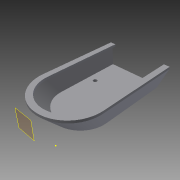
# Autodesk Inventor part: Robot Cover 1
Saved by Autodesk Inventor 2015 SP1 (Build 190203100, 203)
## iProperties
Created: 2017-06-09
Part Number: Robot Cover 1
Material: Generic
Document SubType Name: Modeling
Designer: 0301546
Density: 1 g/cm^3
Appearance: Default
Author: 0301546
Autodesk Inventor part; units mm, degrees
ref_plane "YZ Plane" through (0, 0, 0) normal (1, 0, 0) x (0, 1, 0)
ref_plane "XZ Plane" through (0, 0, 0) normal (0, 1, 0) x (-1, 0, 0)
sketch "Sketch1" plane through (0, 0, 0) normal (0, 1, 0) x (-1, 0, 0)
  line L0 (0, 0) -> (80, 0)
  line L1 (80, 0) -> (80, 100)
  line L2 (80, 100) -> (0, 100)
  line L3 (0, 100) -> (0, 0)
  arc A0 (80, 100) -> (0, 100) centre (40, 100) ccw
  dimension "d0" = 80
  dimension "d1" = 100
  constraints: 8 end point, 2 parallel, 2 point on circle, 1 centre point, 1 horizontal, 1 midpoint, 1 perpendicular
  measures "d0" distance of L0.start L0.end
  measures "d1" distance of L0.end L1.end
extrude "Extrusion1" add sketch "Sketch1" along normal blind 3
sketch3d "3D Sketch1"
ref_plane "Work Plane1" through (-7, -20, 0) normal (0, -1, 0.0000001) x (0, 0.0000001, 1)
sketch "Sketch8" plane through (-7, -20, 0) normal (0, -1, 0.0000001) x (0, 0.0000001, 1)
  line L0 (7.000002, 0) -> (7.000002, 66)
  line L1 (7.000002, 66) -> (87.000002, 66)
  line L2 (87.000002, 66) -> (87.000002, 0)
  line L3 (87.000002, 0) -> (7.000002, 0)
  line L4 (0.000002, -7) -> (0.000002, 73)
  line L5 (100.000002, -7) -> (0.000002, -7)
  line L6 (0.000002, 73) -> (100.000002, 73)
  line L7 (87.000002, 0) -> (87.000002, -7)
  line L8 (87.000002, 66) -> (87.000002, 73)
  line L9 (7.000002, 66) -> (0.000002, 66)
  arc A0 (87.000002, 0) -> (87.000002, 66) centre (87.000002, 33) ccw
  dimension "d24" = 7
  dimension "d25" = 7
  dimension "d26" = 7
  dimension "d27" = 80
  constraints: 14 end point, 4 parallel, 3 perpendicular, 3 point on line, 2 point on circle, 1 centre point, 1 collinear, 1 midpoint
  measures "d24" distance of L1.end L8.end
  measures "d25" distance of L2.end L7.end
  measures "d26" distance of L0.end L9.end
  measures "d27" distance of L0.end L1.end
extrude "Extrusion3" add sketch "Sketch8" along normal blind 3 contours L0 L1 L2 L3 | L2 A0
sketch "Sketch11" plane through (-7, -20, 0) normal (0, 1, -0.0000001) x (1, 0, 0)
  arc A0 (-66, -87.000002) -> (0, -87.000002) centre (-33, -87.000002) ccw
  line L0 (0, -87.000002) -> (0, -7.000002)
  line L1 (0, -87.000002) -> (-3, -87.000002)
  arc A1 (-66, -87.000002) -> (0, -87.000002) centre (-33, -87.000002) ccw
  line L2 (-3, -87.000002) -> (-3, -10.000002)
  line L3 (-63, -87.000002) -> (-63, -10.000002)
  line L4 (-66, -7.000002) -> (0, -7.000002)
  line L5 (-66, -87.000002) -> (-66, -7.000002)
  arc A2 (-63, -87.000002) -> (-3, -87.000002) centre (-33, -87.000002) ccw
  line L6 (-3, -87.000002) -> (-63, -87.000002)
  line L7 (-63, -87.000002) -> (-66, -87.000002)
  line L8 (0, -7.000002) -> (0, -87.000002)
  line L9 (-66, -87.000002) -> (-66, -7.000002)
  line L10 (-66, -7.000002) -> (0, -7.000002)
  line L11 (-66, -7.000002) -> (0, -7.000002)
  line L12 (-3, -10.000002) -> (-3, -7.000002)
  line L13 (-63, -10.000002) -> (-63, -7.000002)
  line L14 (-3, -7.000002) -> (-3, 12.999998)
  line L15 (-3, 12.999998) -> (-63, 12.999998)
  line L16 (-63, 12.999998) -> (-63, -7.000002)
  dimension "d63" = 3
  dimension "d66" = 20
  constraints: 26 end point, 5 collinear, 4 point on circle, 3 horizontal, 3 point on line, 2 centre point, 2 coincident, 2 parallel, 2 tangent, 1 perpendicular, 1 vertical
  measures "d63" distance of L0.start L1.end
  measures "d66" distance of L15.end L13.end
loft "Loft1" add section 1 edges at (-40, 0, 140) (-80, 0, 50) (-40, 0, 0) (0, 0, 50) section 2 edges at (-40, -22.999985, 120.000003) (-73, -22.999994, 47.000003) (-40, -22.999999, 7.000003) (-7, -22.999994, 47.000003)
sketch "Sketch12" plane through (0, 0, 0) normal (0, -1, 0) x (1, 0, 0)
  line L0 (-77, 3) -> (-3, 3)
  line L1 (-3, 3) -> (-3, 100)
  line L2 (-3, 100) -> (-77, 100)
  line L3 (-77, 100) -> (-77, 3)
  line L4 (-77, 3) -> (-77, 0)
  line L5 (0, 0) -> (-80, 0) projected
  line L6 (-3, 3) -> (0, 3)
  line L7 (-77, 3) -> (-80, 3)
  line L8 (-80, 0) -> (-80, 100) projected
  line L9 (0, 100) -> (0, 0) projected
  arc A0 (0, 100) -> (-80, 100) centre (-40, 100) ccw projected
  circle A1 centre (-40, 100) radius 37
  line L10 (-3, 3) -> (-3, 0)
  line L11 (-77, -17) -> (-3, -17)
  line L12 (-3, -17) -> (-3, 3)
  line L13 (-77, -17) -> (-77, 3)
  dimension "d49" = 3
  dimension "d50" = 3
  dimension "d51" = 3
  dimension "d65" = 20
  constraints: 22 end point, 4 collinear, 4 parallel, 4 point on line, 2 perpendicular, 1 coincident, 1 horizontal, 1 horizontal alignment, 1 midpoint, 2 other
  measures "d49" distance of L0.end L6.end
  measures "d50" distance of L0.start L4.end
  measures "d51" distance of L0.start L7.end
  measures "d65" distance of L11.end L0.end
loft "Loft2" cut profiles "Sketch12", "Sketch11" contours L3 A1 L1 L0 | L0 L10 L5 L4 | A1 L2 | L2 A1 | L5 L12 L11 L13 / L6 A2 | L3 L13 L4 L12 L2 L6 | L16 L15 L14 L4
sketch "Sketch13" plane through (0, 3, 0) normal (0, 1, 0) x (1, 0, 0)
  line L0 (-73, -100) -> (-73, -7)
  line L1 (-73, -7) -> (-7, -7)
  line L2 (-7, -7) -> (-7, -100)
  line L3 (-7, -100) -> (-73, -100)
  line L4 (-73, -7) -> (-73, 0)
  line L5 (-73, -7) -> (-80, -7)
  line L6 (-80, 0) -> (-80, -100) projected
  line L7 (-7, -7) -> (0, -7)
  line L8 (-80, 0) -> (-80, -100) projected
  line L9 (0, -100) -> (0, 0) projected
  line L10 (0, 0) -> (-80, 0) projected
  circle A0 centre (-40, -100) radius 33
  line L11 (-7, -7) -> (-7, 0)
  dimension "d57" = 7
  dimension "d58" = 7
  dimension "d59" = 7
  dimension "d60" = 93
  constraints: 16 end point, 6 point on line, 3 parallel, 2 perpendicular, 2 vertical, 1 horizontal, 1 horizontal alignment, 1 midpoint, 2 other
  measures "d57" distance of L0.end L5.end
  measures "d58" distance of L1.end L7.end
  measures "d59" distance of L0.end L4.end
  measures "d60" distance of L0.start L0.end
extrude "Extrusion4" cut sketch "Sketch13" against normal blind 3 contours A0 L3 | L0 L1 L2 A0 | L3 A0 | L4 L10 L11 L1
sketch3d "3D Sketch2"
ref_plane "Work Plane2" through (-40, -4.999994, 150.000001) normal (0, 0.0000001, 1) x (1, 0, 0)
sketch "Sketch14" plane through (-40, -4.999994, 150.000001) normal (0, 0.0000001, 1) x (1, 0, 0)
  ellipse E0 centre (0, 5) end of major axis (-37, 5) minor radius 0.000005 (-37, 5) -> (37, 5) ccw
  line L0 (0, 5) -> (0, 0)
  line L1 (0, 0) -> (-2.7, 0)
  circle A0 centre (0, 0) radius 2.7
  point P0 (40, 5.000012)
  dimension "d76" = 5
  dimension "d77" = 2.7
  constraints: 4 end point, 1 coincident, 1 horizontal, 1 horizontal alignment, 1 vertical, 3 other
  measures "d76" distance of L0.start L0.end
  measures "d77" distance of L0.end L1.end
extrude "Extrusion5" cut sketch "Sketch14" against normal blind 21.75
sketch "Sketch15" plane through (-40, -4.999994, 150.000001) normal (0, 0.0000001, 1) x (1, 0, 0)
  point P0 (40, 5.000012)
sketch "Sketch16" plane through (-7, -23, 0) normal (0, -1, 0.0000001) x (1, 0, 0)
  line L0 (0, 87.000002) -> (0, 7.000002)
  line L1 (0, 7.000002) -> (-66, 7.000002)
  line L2 (-66, 7.000002) -> (-66, 87.000002)
  line L3 (-66, 87.000002) -> (-66, 7.000002)
  line L4 (-66, 7.000002) -> (0, 7.000002)
  line L5 (0, 7.000002) -> (0, 87.000002)
  line L6 (0, 47.000002) -> (-13, 47.000002)
  line L7 (-66, 47.000002) -> (-53, 47.000002)
  circle A0 centre (-13, 47.000002) radius 2.7
  circle A1 centre (-53, 47.000002) radius 2.7
  point P0 (7, 0.000002)
  dimension "d78" = 13
  dimension "d79" = 13
  dimension "d80" = 5.4
  dimension "d81" = 5.4
  constraints: 10 end point, 3 midpoint, 2 centre point, 2 coincident, 2 collinear, 2 horizontal, 1 perpendicular, 1 vertical
  measures "d78" distance of L6.start L6.end
  measures "d79" distance of L7.start L7.end
  measures "d80" diameter of A0
  measures "d81" diameter of A1
extrude "Extrusion6" cut sketch "Sketch16" against normal blind 21.75
sketch "Sketch18" plane through (-7, -23, 0) normal (0, -1, 0.0000001) x (1, 0, 0)
  arc A0 (0, 87.000002) -> (-66, 87.000002) centre (-33, 87.000002) ccw
  circle A1 centre (-33, 87.000002) radius 33
  line L0 (-2.41471, 89.14761) -> (-2.446153, 88.174292)
  line L1 (-2.446153, 88.174292) -> (-7.698114, 88.343958)
  line L2 (-7.698114, 88.343958) -> (-4.18744, 86.326392)
  line L3 (-4.18744, 86.326392) -> (-4.206593, 85.733508)
  line L4 (-4.206593, 85.733508) -> (-7.839688, 83.96156)
  line L5 (-7.839688, 83.96156) -> (-2.587727, 83.791895)
  line L6 (-2.587727, 83.791895) -> (-2.617096, 82.882806)
  line L7 (-2.617096, 82.882806) -> (-8.713915, 83.079765)
  line L8 (-8.713915, 83.079765) -> (-8.67114, 84.403872)
  line L9 (-8.67114, 84.403872) -> (-5.217825, 86.122278)
  line L10 (-5.217825, 86.122278) -> (-8.555103, 87.995758)
  line L11 (-8.555103, 87.995758) -> (-8.51153, 89.344569)
  line L12 (-8.51153, 89.344569) -> (-2.41471, 89.14761)
  spline S0 degree 2 poles (-5.708587, 94.553393) (-4.57126, 94.764353) (-3.088451, 93.681946) (-2.886507, 92.593223) knots 0 0 0 1 2 2 2
  spline S1 degree 2 poles (-2.886507, 92.593223) (-2.67735, 91.465617) (-3.716719, 89.940515) (-4.815163, 89.736767) knots 0 0 0 1 2 2 2
  spline S2 degree 2 poles (-4.815163, 89.736767) (-5.942768, 89.527611) (-7.438003, 90.622796) (-7.639947, 91.711519) knots 0 0 0 1 2 2 2
  spline S3 degree 2 poles (-7.639947, 91.711519) (-7.841892, 92.800241) (-6.841053, 94.343335) (-5.708587, 94.553393) knots 0 0 0 1 2 2 2
  spline S4 degree 2 poles (-5.53459, 93.615342) (-6.409456, 93.453065) (-7.118479, 92.532218) (-6.987756, 91.827464) knots 0 0 0 1 2 2 2
  spline S5 degree 2 poles (-6.987756, 91.827464) (-6.857033, 91.122711) (-5.864026, 90.512542) (-4.989159, 90.674819) knots 0 0 0 1 2 2 2
  spline S6 degree 2 poles (-4.989159, 90.674819) (-4.138595, 90.832588) (-3.406171, 91.762803) (-3.536894, 92.467557) knots 0 0 0 1 2 2 2
  spline S7 degree 2 poles (-3.536894, 92.467557) (-3.666716, 93.16745) (-4.669444, 93.775816) (-5.53459, 93.615342) knots 0 0 0 1 2 2 2
  line L13 (-5.265037, 99.868285) -> (-4.935567, 99.004601)
  line L14 (-4.935567, 99.004601) -> (-5.406668, 98.82489)
  spline S8 degree 2 poles (-5.406668, 98.82489) (-4.964173, 98.538685) (-4.389111, 97.9327) (-4.221733, 97.49393) knots 0 0 0 1 2 2 2
  spline S9 degree 2 poles (-4.221733, 97.49393) (-4.093117, 97.156769) (-4.052343, 96.495109) (-4.166375, 96.197655) knots 0 0 0 1 2 2 2
  spline S10 degree 2 poles (-4.166375, 96.197655) (-4.282168, 95.904819) (-4.79383, 95.429226) (-5.227982, 95.263611) knots 0 0 0 1 2 2 2
  line L15 (-5.227982, 95.263611) -> (-8.003781, 94.204728)
  line L16 (-8.003781, 94.204728) -> (-8.33325, 95.068413)
  line L17 (-8.33325, 95.068413) -> (-5.894612, 95.998679)
  spline S11 degree 2 poles (-5.894612, 95.998679) (-5.552833, 96.129057) (-5.12773, 96.360001) (-5.001982, 96.529656) knots 0 0 0 1 2 2 2
  spline S12 degree 2 poles (-5.001982, 96.529656) (-4.876234, 96.699312) (-4.861245, 97.117707) (-4.991623, 97.459486) knots 0 0 0 1 2 2 2
  spline S13 degree 2 poles (-4.991623, 97.459486) (-5.11143, 97.773553) (-5.68473, 98.37492) (-6.016328, 98.592324) knots 0 0 0 1 2 2 2
  line L18 (-6.016328, 98.592324) -> (-9.212422, 97.373111)
  line L19 (-9.212422, 97.373111) -> (-9.541892, 98.236796)
  line L20 (-9.541892, 98.236796) -> (-5.265037, 99.868285)
  line L21 (-8.098287, 104.745318) -> (-7.616799, 103.956223)
  line L22 (-7.616799, 103.956223) -> (-9.844832, 102.596729)
  spline S14 degree 2 poles (-9.844832, 102.596729) (-10.114896, 102.431942) (-10.540448, 102.085418) (-10.625629, 101.911834) knots 0 0 0 1 2 2 2
  spline S15 degree 2 poles (-10.625629, 101.911834) (-10.7141, 101.724662) (-10.649013, 101.295318) (-10.466203, 100.995715) knots 0 0 0 1 2 2 2
  spline S16 degree 2 poles (-10.466203, 100.995715) (-10.288541, 100.704552) (-9.645846, 100.239665) (-9.252047, 100.068802) knots 0 0 0 1 2 2 2
  line L23 (-9.252047, 100.068802) -> (-6.331974, 101.850563)
  line L24 (-6.331974, 101.850563) -> (-5.850487, 101.061469)
  line L25 (-5.850487, 101.061469) -> (-9.757984, 98.677204)
  line L26 (-9.757984, 98.677204) -> (-10.239471, 99.466299)
  line L27 (-10.239471, 99.466299) -> (-9.804836, 99.731504)
  spline S17 degree 2 poles (-9.804836, 99.731504) (-10.286964, 99.923751) (-10.98516, 100.441635) (-11.216892, 100.821413) knots 0 0 0 1 2 2 2
  spline S18 degree 2 poles (-11.216892, 100.821413) (-11.639159, 101.513454) (-11.355941, 102.757573) (-10.634362, 103.197864) knots 0 0 0 1 2 2 2
  line L28 (-10.634362, 103.197864) -> (-8.098287, 104.745318)
  spline S19 degree 2 poles (-9.913482, 107.077714) (-9.429309, 106.496682) (-9.438824, 105.388437) (-10.035046, 104.891606) knots 0 0 0 1 2 2 2
  line L29 (-10.035046, 104.891606) -> (-11.98321, 103.2682)
  line L30 (-11.98321, 103.2682) -> (-11.584479, 102.789704)
  line L31 (-11.584479, 102.789704) -> (-12.074368, 102.381479)
  line L32 (-12.074368, 102.381479) -> (-12.473099, 102.859976)
  line L33 (-12.473099, 102.859976) -> (-13.483258, 102.01821)
  line L34 (-13.483258, 102.01821) -> (-14.075026, 102.72836)
  line L35 (-14.075026, 102.72836) -> (-13.064867, 103.570125)
  line L36 (-13.064867, 103.570125) -> (-14.153466, 104.876496)
  line L37 (-14.153466, 104.876496) -> (-13.663577, 105.284721)
  line L38 (-13.663577, 105.284721) -> (-12.574978, 103.97835)
  line L39 (-12.574978, 103.97835) -> (-10.90024, 105.373909)
  spline S20 degree 2 poles (-10.90024, 105.373909) (-10.634409, 105.595426) (-10.360982, 105.86188) (-10.298952, 106.042262) knots 0 0 0 1 2 2 2
  spline S21 degree 2 poles (-10.298952, 106.042262) (-10.242619, 106.198592) (-10.369828, 106.575183) (-10.575523, 106.822026) knots 0 0 0 1 2 2 2
  spline S22 degree 2 poles (-10.575523, 106.822026) (-10.721092, 106.996716) (-11.077421, 107.246726) (-11.164131, 107.296729) knots 0 0 0 1 2 2 2
  line L40 (-11.164131, 107.296729) -> (-11.19894, 107.338502)
  line L41 (-11.19894, 107.338502) -> (-10.667278, 107.781537)
  spline S23 degree 2 poles (-10.667278, 107.781537) (-10.453987, 107.618239) (-10.059051, 107.252403) (-9.913482, 107.077714) knots 0 0 0 1 2 2 2
  line L42 (-18.059872, 113.792399) -> (-17.031002, 113.064131)
  line L43 (-17.031002, 113.064131) -> (-16.540962, 109.743609)
  line L44 (-16.540962, 109.743609) -> (-15.633136, 109.101019)
  line L45 (-15.633136, 109.101019) -> (-14.230862, 111.082098)
  line L46 (-14.230862, 111.082098) -> (-13.43601, 110.519475)
  line L47 (-13.43601, 110.519475) -> (-16.960258, 105.540552)
  line L48 (-16.960258, 105.540552) -> (-18.501545, 106.631526)
  spline S24 degree 2 poles (-18.501545, 106.631526) (-19.013963, 106.994233) (-19.642259, 107.578257) (-19.832987, 107.967626) knots 0 0 0 1 2 2 2
  spline S25 degree 2 poles (-19.832987, 107.967626) (-20.02775, 108.359852) (-20.016751, 109.145444) (-19.739723, 109.536818) knots 0 0 0 1 2 2 2
  spline S26 degree 2 poles (-19.739723, 109.536818) (-19.354169, 110.081514) (-18.16579, 110.348647) (-17.467189, 110.120632) knots 0 0 0 1 2 2 2
  line L49 (-17.467189, 110.120632) -> (-18.059872, 113.792399)
  spline S27 degree 2 poles (-18.875465, 109.0038) (-19.029686, 108.785922) (-19.081131, 108.319661) (-18.968607, 108.076492) knots 0 0 0 1 2 2 2
  spline S28 degree 2 poles (-18.968607, 108.076492) (-18.864833, 107.863741) (-18.4672, 107.467214) (-18.136348, 107.233025) knots 0 0 0 1 2 2 2
  line L50 (-18.136348, 107.233025) -> (-17.349565, 106.676114)
  line L51 (-17.349565, 106.676114) -> (-16.024402, 108.548254)
  line L52 (-16.024402, 108.548254) -> (-16.722419, 109.042334)
  spline S29 degree 2 poles (-16.722419, 109.042334) (-17.065376, 109.28509) (-17.681471, 109.569774) (-17.982488, 109.546648) knots 0 0 0 1 2 2 2
  spline S30 degree 2 poles (-17.982488, 109.546648) (-18.253086, 109.532271) (-18.692684, 109.262026) (-18.875465, 109.0038) knots 0 0 0 1 2 2 2
  spline S31 degree 2 poles (-23.608454, 113.714677) (-23.131869, 114.76866) (-21.396378, 115.367327) (-20.387436, 114.911109) knots 0 0 0 1 2 2 2
  spline S32 degree 2 poles (-20.387436, 114.911109) (-19.342461, 114.438597) (-18.684496, 112.714269) (-19.144787, 111.696318) knots 0 0 0 1 2 2 2
  spline S33 degree 2 poles (-19.144787, 111.696318) (-19.617299, 110.651343) (-21.370376, 110.049778) (-22.379317, 110.505997) knots 0 0 0 1 2 2 2
  spline S34 degree 2 poles (-22.379317, 110.505997) (-23.388259, 110.962215) (-24.083002, 112.665197) (-23.608454, 113.714677) knots 0 0 0 1 2 2 2
  spline S35 degree 2 poles (-22.739142, 113.321596) (-23.105746, 112.510839) (-22.755007, 111.402843) (-22.101897, 111.107523) knots 0 0 0 1 2 2 2
  spline S36 degree 2 poles (-22.101897, 111.107523) (-21.448787, 110.812203) (-20.380703, 111.278642) (-20.014099, 112.089399) knots 0 0 0 1 2 2 2
  spline S37 degree 2 poles (-20.014099, 112.089399) (-19.657678, 112.877635) (-20.002739, 114.010189) (-20.655848, 114.305508) knots 0 0 0 1 2 2 2
  spline S38 degree 2 poles (-20.655848, 114.305508) (-21.304454, 114.598792) (-22.376612, 114.123344) (-22.739142, 113.321596) knots 0 0 0 1 2 2 2
  line L53 (-28.900006, 112.716014) -> (-24.472723, 118.039089)
  line L54 (-24.472723, 118.039089) -> (-23.515652, 117.791192)
  line L55 (-23.515652, 117.791192) -> (-24.946378, 116.190702)
  line L56 (-24.946378, 116.190702) -> (-24.105079, 111.474051)
  line L57 (-24.105079, 111.474051) -> (-25.066936, 111.723187)
  line L58 (-25.066936, 111.723187) -> (-25.671399, 115.382745)
  line L59 (-25.671399, 115.382745) -> (-27.966862, 112.474314)
  line L60 (-27.966862, 112.474314) -> (-28.900006, 112.716014)
  spline S39 degree 2 poles (-31.529156, 116.999221) (-31.409984, 117.0585) (-31.014623, 117.272795) (-30.831001, 117.33153) knots 0 0 0 1 2 2 2
  spline S40 degree 2 poles (-30.831001, 117.33153) (-30.575479, 117.418853) (-30.112671, 117.493433) (-29.703868, 117.458515) knots 0 0 0 1 2 2 2
  spline S41 degree 2 poles (-29.703868, 117.458515) (-29.36402, 117.429488) (-28.776292, 117.165954) (-28.561208, 116.954093) knots 0 0 0 1 2 2 2
  spline S42 degree 2 poles (-28.561208, 116.954093) (-28.360479, 116.74842) (-28.141628, 116.174064) (-28.167711, 115.868693) knots 0 0 0 1 2 2 2
  spline S43 degree 2 poles (-28.167711, 115.868693) (-28.208097, 115.395861) (-28.743068, 114.766821) (-29.281561, 114.619326) knots 0 0 0 1 2 2 2
  spline S44 degree 2 poles (-29.281561, 114.619326) (-29.754763, 114.481138) (-31.017158, 114.455008) (-31.744128, 114.482372) knots 0 0 0 1 2 2 2
  line L61 (-31.744128, 114.482372) -> (-31.756748, 114.334612)
  spline S45 degree 2 poles (-31.756748, 114.334612) (-31.779466, 114.068643) (-31.610638, 113.721818) (-31.446244, 113.613512) knots 0 0 0 1 2 2 2
  spline S46 degree 2 poles (-31.446244, 113.613512) (-31.276925, 113.504786) (-30.769738, 113.401931) (-30.503769, 113.379213) knots 0 0 0 1 2 2 2
  spline S47 degree 2 poles (-30.503769, 113.379213) (-30.183622, 113.351869) (-29.308226, 113.435859) (-28.86668, 113.551945) knots 0 0 0 1 2 2 2
  line L62 (-28.86668, 113.551945) -> (-28.812501, 113.547317)
  line L63 (-28.812501, 113.547317) -> (-28.87939, 112.764188)
  spline S48 degree 2 poles (-28.87939, 112.764188) (-29.140556, 112.72696) (-30.103768, 112.660392) (-30.56675, 112.699937) knots 0 0 0 1 2 2 2
  spline S49 degree 2 poles (-30.56675, 112.699937) (-31.133164, 112.748316) (-31.893822, 112.962124) (-32.187711, 113.180716) knots 0 0 0 1 2 2 2
  spline S50 degree 2 poles (-32.187711, 113.180716) (-32.467246, 113.39312) (-32.711863, 114.014328) (-32.675263, 114.442832) knots 0 0 0 1 2 2 2
  line L64 (-32.675263, 114.442832) -> (-32.408967, 117.560573)
  line L65 (-32.408967, 117.560573) -> (-31.487929, 117.481904)
  line L66 (-31.487929, 117.481904) -> (-31.529156, 116.999221)
  line L67 (-31.583846, 116.358927) -> (-31.691962, 115.093114)
  spline S51 degree 2 poles (-31.691962, 115.093114) (-31.364786, 115.089975) (-30.352865, 115.087886) (-30.040763, 115.140609) knots 0 0 0 1 2 2 2
  spline S52 degree 2 poles (-30.040763, 115.140609) (-29.66337, 115.202638) (-29.152377, 115.550934) (-29.122929, 115.895707) knots 0 0 0 1 2 2 2
  spline S53 degree 2 poles (-29.122929, 115.895707) (-29.089274, 116.289735) (-29.58221, 116.733701) (-30.08952, 116.777032) knots 0 0 0 1 2 2 2
  spline S54 degree 2 poles (-30.08952, 116.777032) (-30.527875, 116.814473) (-31.258702, 116.564335) (-31.583846, 116.358927) knots 0 0 0 1 2 2 2
  line L68 (-34.644676, 117.459134) -> (-33.720979, 117.494983)
  line L69 (-33.720979, 117.494983) -> (-33.47387, 111.127896)
  line L70 (-33.47387, 111.127896) -> (-34.397567, 111.092047)
  line L71 (-34.397567, 111.092047) -> (-34.644676, 117.459134)
  line L72 (-39.181257, 116.939493) -> (-37.544054, 111.063307)
  line L73 (-37.544054, 111.063307) -> (-41.953574, 109.834741)
  line L74 (-41.953574, 109.834741) -> (-42.147279, 110.529979)
  line L75 (-42.147279, 110.529979) -> (-38.675853, 111.497176)
  line L76 (-38.675853, 111.497176) -> (-39.124293, 113.106699)
  line L77 (-39.124293, 113.106699) -> (-42.357624, 112.205839)
  line L78 (-42.357624, 112.205839) -> (-42.551329, 112.901076)
  line L79 (-42.551329, 112.901076) -> (-39.317998, 113.801936)
  line L80 (-39.317998, 113.801936) -> (-39.925647, 115.982887)
  line L81 (-39.925647, 115.982887) -> (-43.397073, 115.01569)
  line L82 (-43.397073, 115.01569) -> (-43.590778, 115.710927)
  line L83 (-43.590778, 115.710927) -> (-39.181257, 116.939493)
  line L84 (-45.349615, 114.891769) -> (-44.498796, 115.253167)
  line L85 (-44.498796, 115.253167) -> (-42.007662, 109.388433)
  line L86 (-42.007662, 109.388433) -> (-42.85848, 109.027035)
  line L87 (-42.85848, 109.027035) -> (-45.349615, 114.891769)
  spline S55 degree 2 poles (-48.711561, 113.265994) (-47.578612, 113.923598) (-45.708056, 113.586141) (-45.137306, 112.602828) knots 0 0 0 1 2 2 2
  spline S56 degree 2 poles (-45.137306, 112.602828) (-44.576481, 111.636615) (-45.12561, 109.786088) (-46.104649, 109.217818) knots 0 0 0 1 2 2 2
  spline S57 degree 2 poles (-46.104649, 109.217818) (-46.549277, 108.95974) (-47.348847, 108.781422) (-47.736885, 108.85912) knots 0 0 0 1 2 2 2
  spline S58 degree 2 poles (-47.736885, 108.85912) (-48.120647, 108.9393) (-48.773938, 109.4346) (-49.049387, 109.909155) knots 0 0 0 1 2 2 2
  line L88 (-49.049387, 109.909155) -> (-49.260317, 110.272554)
  line L89 (-49.260317, 110.272554) -> (-45.976905, 112.178366)
  spline S59 degree 2 poles (-45.976905, 112.178366) (-46.37643, 112.866685) (-47.630175, 113.116341) (-48.365523, 112.689519) knots 0 0 0 1 2 2 2
  spline S60 degree 2 poles (-48.365523, 112.689519) (-48.63059, 112.535664) (-49.077997, 112.144513) (-49.234268, 111.950926) knots 0 0 0 1 2 2 2
  spline S61 degree 2 poles (-49.234268, 111.950926) (-49.402676, 111.738863) (-49.610817, 111.418003) (-49.669444, 111.292523) knots 0 0 0 1 2 2 2
  line L90 (-49.669444, 111.292523) -> (-49.716472, 111.265227)
  line L91 (-49.716472, 111.265227) -> (-50.138331, 111.992024)
  spline S62 degree 2 poles (-50.138331, 111.992024) (-50.024544, 112.120942) (-49.689251, 112.498459) (-49.544849, 112.633716) knots 0 0 0 1 2 2 2
  spline S63 degree 2 poles (-49.544849, 112.633716) (-49.346244, 112.823297) (-48.998004, 113.099731) (-48.711561, 113.265994) knots 0 0 0 1 2 2 2
  spline S64 degree 2 poles (-48.186915, 110.215434) (-48.022029, 109.951054) (-47.656919, 109.637138) (-47.456009, 109.576568) knots 0 0 0 1 2 2 2
  spline S65 degree 2 poles (-47.456009, 109.576568) (-47.228071, 109.508824) (-46.700177, 109.603754) (-46.375256, 109.79235) knots 0 0 0 1 2 2 2
  spline S66 degree 2 poles (-46.375256, 109.79235) (-46.058885, 109.975983) (-45.706073, 110.392247) (-45.611571, 110.652863) knots 0 0 0 1 2 2 2
  spline S67 degree 2 poles (-45.611571, 110.652863) (-45.528101, 110.912791) (-45.560845, 111.402477) (-45.681603, 111.669608) knots 0 0 0 1 2 2 2
  line L92 (-45.681603, 111.669608) -> (-48.186915, 110.215434)
  spline S68 degree 2 poles (-52.84998, 110.299114) (-52.414795, 110.657141) (-51.500375, 111.031768) (-51.052355, 111.016284) knots 0 0 0 1 2 2 2
  spline S69 degree 2 poles (-51.052355, 111.016284) (-50.603658, 111.007758) (-49.745764, 110.548534) (-49.362612, 110.08281) knots 0 0 0 1 2 2 2
  spline S70 degree 2 poles (-49.362612, 110.08281) (-48.979459, 109.617086) (-48.718191, 108.69262) (-48.781704, 108.256296) knots 0 0 0 1 2 2 2
  spline S71 degree 2 poles (-48.781704, 108.256296) (-48.842077, 107.816155) (-49.382333, 106.955607) (-49.809883, 106.603861) knots 0 0 0 1 2 2 2
  spline S72 degree 2 poles (-49.809883, 106.603861) (-50.161085, 106.314926) (-50.941273, 105.948314) (-51.284976, 105.844782) knots 0 0 0 1 2 2 2
  line L93 (-51.284976, 105.844782) -> (-51.83458, 106.512828)
  line L94 (-51.83458, 106.512828) -> (-51.792589, 106.547375)
  spline S73 degree 2 poles (-51.792589, 106.547375) (-51.672272, 106.556743) (-51.322531, 106.614033) (-51.091077, 106.682829) knots 0 0 0 1 2 2 2
  spline S74 degree 2 poles (-51.091077, 106.682829) (-50.891948, 106.744234) (-50.412605, 106.978561) (-50.225552, 107.13245) knots 0 0 0 1 2 2 2
  spline S75 degree 2 poles (-50.225552, 107.13245) (-49.672028, 107.587837) (-49.574892, 108.839167) (-50.099372, 109.476675) knots 0 0 0 1 2 2 2
  spline S76 degree 2 poles (-50.099372, 109.476675) (-50.611289, 110.098913) (-51.834978, 110.263597) (-52.411406, 109.789368) knots 0 0 0 1 2 2 2
  spline S77 degree 2 poles (-52.411406, 109.789368) (-52.758791, 109.503573) (-53.190806, 108.744878) (-53.281231, 108.356827) knots 0 0 0 1 2 2 2
  line L95 (-53.281231, 108.356827) -> (-53.323222, 108.322281)
  line L96 (-53.323222, 108.322281) -> (-53.872827, 108.990327)
  spline S78 degree 2 poles (-53.872827, 108.990327) (-53.800486, 109.120256) (-53.580999, 109.499265) (-53.473191, 109.632767) knots 0 0 0 1 2 2 2
  spline S79 degree 2 poles (-53.473191, 109.632767) (-53.327643, 109.829324) (-53.079024, 110.110678) (-52.84998, 110.299114) knots 0 0 0 1 2 2 2
  spline S80 degree 2 poles (-55.795106, 107.407965) (-55.278857, 107.960693) (-54.178045, 108.089192) (-53.610867, 107.559446) knots 0 0 0 1 2 2 2
  line L97 (-53.610867, 107.559446) -> (-51.757602, 105.828494)
  line L98 (-51.757602, 105.828494) -> (-51.332456, 106.283681)
  line L99 (-51.332456, 106.283681) -> (-50.866431, 105.848412)
  line L100 (-50.866431, 105.848412) -> (-51.291577, 105.393225)
  line L101 (-51.291577, 105.393225) -> (-50.330625, 104.495694)
  line L102 (-50.330625, 104.495694) -> (-50.961596, 103.820137)
  line L103 (-50.961596, 103.820137) -> (-51.922548, 104.717668)
  line L104 (-51.922548, 104.717668) -> (-53.083265, 103.474933)
  line L105 (-53.083265, 103.474933) -> (-53.54929, 103.910202)
  line L106 (-53.54929, 103.910202) -> (-52.388574, 105.152937)
  line L107 (-52.388574, 105.152937) -> (-53.981731, 106.640949)
  spline S81 degree 2 poles (-53.981731, 106.640949) (-54.234613, 106.877142) (-54.533028, 107.115278) (-54.719728, 107.154373) knots 0 0 0 1 2 2 2
  spline S82 degree 2 poles (-54.719728, 107.154373) (-54.881854, 107.19081) (-55.239683, 107.017716) (-55.459004, 106.782897) knots 0 0 0 1 2 2 2
  spline S83 degree 2 poles (-55.459004, 106.782897) (-55.614216, 106.616718) (-55.817932, 106.23204) (-55.856753, 106.139782) knots 0 0 0 1 2 2 2
  line L108 (-55.856753, 106.139782) -> (-55.893869, 106.100043)
  line L109 (-55.893869, 106.100043) -> (-56.399633, 106.572428)
  spline S84 degree 2 poles (-56.399633, 106.572428) (-56.264153, 106.804386) (-55.950318, 107.241785) (-55.795106, 107.407965) knots 0 0 0 1 2 2 2
  line L110 (-55.553037, 101.488777) -> (-55.523642, 101.528521)
  spline S85 degree 2 poles (-55.523642, 101.528521) (-55.442041, 101.597284) (-55.298875, 101.774224) (-55.201872, 101.905377) knots 0 0 0 1 2 2 2
  spline S86 degree 2 poles (-55.201872, 101.905377) (-54.97847, 102.207426) (-54.762012, 102.9573) (-54.77968, 103.382313) knots 0 0 0 1 2 2 2
  line L111 (-54.77968, 103.382313) -> (-57.390816, 105.313563)
  line L112 (-57.390816, 105.313563) -> (-56.841129, 106.056763)
  line L113 (-56.841129, 106.056763) -> (-53.160899, 103.334788)
  line L114 (-53.160899, 103.334788) -> (-53.710585, 102.591588)
  line L115 (-53.710585, 102.591588) -> (-54.259042, 102.997239)
  spline S87 degree 2 poles (-54.259042, 102.997239) (-54.256822, 102.368455) (-54.457217, 101.582108) (-54.668861, 101.295956) knots 0 0 0 1 2 2 2
  spline S88 degree 2 poles (-54.668861, 101.295956) (-54.751167, 101.184675) (-54.844361, 101.075298) (-54.909195, 101.012579) knots 0 0 0 1 2 2 2
  line L116 (-54.909195, 101.012579) -> (-55.553037, 101.488777)
  spline S89 degree 2 poles (-59.064586, 98.068529) (-60.086189, 98.611063) (-60.573474, 100.381058) (-60.054126, 101.359003) knots 0 0 0 1 2 2 2
  spline S90 degree 2 poles (-60.054126, 101.359003) (-59.516229, 102.371874) (-57.75361, 102.919047) (-56.766933, 102.395061) knots 0 0 0 1 2 2 2
  spline S91 degree 2 poles (-56.766933, 102.395061) (-55.754062, 101.857164) (-55.265001, 100.069435) (-55.784349, 99.09149) knots 0 0 0 1 2 2 2
  spline S92 degree 2 poles (-55.784349, 99.09149) (-56.303698, 98.113545) (-58.047349, 97.528314) (-59.064586, 98.068529) knots 0 0 0 1 2 2 2
  spline S93 degree 2 poles (-58.617112, 98.911133) (-57.831264, 98.4938) (-56.703237, 98.773493) (-56.367051, 99.406538) knots 0 0 0 1 2 2 2
  spline S94 degree 2 poles (-56.367051, 99.406538) (-56.030866, 100.039582) (-56.428559, 101.135123) (-57.214408, 101.552457) knots 0 0 0 1 2 2 2
  spline S95 degree 2 poles (-57.214408, 101.552457) (-57.978427, 101.958198) (-59.130601, 101.685731) (-59.466787, 101.052687) knots 0 0 0 1 2 2 2
  spline S96 degree 2 poles (-59.466787, 101.052687) (-59.800654, 100.424008) (-59.394229, 99.32383) (-58.617112, 98.911133) knots 0 0 0 1 2 2 2
  line L117 (-62.730862, 94.14615) -> (-62.45137, 95.027277)
  line L118 (-62.45137, 95.027277) -> (-59.963481, 94.238123)
  spline S97 degree 2 poles (-59.963481, 94.238123) (-59.661919, 94.142468) (-59.121189, 94.048739) (-58.93431, 94.098367) knots 0 0 0 1 2 2 2
  spline S98 degree 2 poles (-58.93431, 94.098367) (-58.735017, 94.15443) (-58.453748, 94.485278) (-58.347631, 94.819823) knots 0 0 0 1 2 2 2
  spline S99 degree 2 poles (-58.347631, 94.819823) (-58.244503, 95.144945) (-58.315439, 95.934974) (-58.444917, 96.34425) knots 0 0 0 1 2 2 2
  line L119 (-58.444917, 96.34425) -> (-61.705559, 97.37852)
  line L120 (-61.705559, 97.37852) -> (-61.426067, 98.259647)
  line L121 (-61.426067, 98.259647) -> (-57.062838, 96.875638)
  line L122 (-57.062838, 96.875638) -> (-57.34233, 95.994511)
  line L123 (-57.34233, 95.994511) -> (-57.827657, 96.148456)
  spline S100 degree 2 poles (-57.827657, 96.148456) (-57.656354, 95.658495) (-57.588989, 94.791809) (-57.723504, 94.367738) knots 0 0 0 1 2 2 2
  spline S101 degree 2 poles (-57.723504, 94.367738) (-57.96862, 93.594984) (-59.093267, 92.992311) (-59.899004, 93.247889) knots 0 0 0 1 2 2 2
  line L124 (-59.899004, 93.247889) -> (-62.730862, 94.14615)
  line L125 (-63.101039, 91.938733) -> (-62.937569, 92.848557)
  line L126 (-62.937569, 92.848557) -> (-58.432241, 92.039073)
  line L127 (-58.432241, 92.039073) -> (-58.595711, 91.12925)
  line L128 (-58.595711, 91.12925) -> (-63.101039, 91.938733)
  line L129 (-57.858683, 90.926512) -> (-57.672484, 91.962835)
  line L130 (-57.672484, 91.962835) -> (-56.884295, 91.821219)
  line L131 (-56.884295, 91.821219) -> (-57.070494, 90.784896)
  line L132 (-57.070494, 90.784896) -> (-57.858683, 90.926512)
  spline S102 degree 2 poles (-63.574589, 88.436928) (-63.538456, 88.999301) (-63.186863, 89.922823) (-62.869324, 90.239257) knots 0 0 0 1 2 2 2
  spline S103 degree 2 poles (-62.869324, 90.239257) (-62.556401, 90.56094) (-61.634804, 90.873236) (-61.032966, 90.834567) knots 0 0 0 1 2 2 2
  spline S104 degree 2 poles (-61.032966, 90.834567) (-60.431127, 90.795898) (-59.577758, 90.354697) (-59.302691, 90.010094) knots 0 0 0 1 2 2 2
  spline S105 degree 2 poles (-59.302691, 90.010094) (-59.022692, 89.665175) (-58.763847, 88.682618) (-58.799347, 88.13011) knots 0 0 0 1 2 2 2
  spline S106 degree 2 poles (-58.799347, 88.13011) (-58.828507, 87.676265) (-59.094197, 86.8562) (-59.25356, 86.534557) knots 0 0 0 1 2 2 2
  line L133 (-59.25356, 86.534557) -> (-60.116853, 86.590025)
  line L134 (-60.116853, 86.590025) -> (-60.113366, 86.644289)
  spline S107 degree 2 poles (-60.113366, 86.644289) (-60.037964, 86.738514) (-59.84072, 87.032956) (-59.732728, 87.248923) knots 0 0 0 1 2 2 2
  spline S108 degree 2 poles (-59.732728, 87.248923) (-59.641437, 87.436243) (-59.484829, 87.946294) (-59.469298, 88.188016) knots 0 0 0 1 2 2 2
  spline S109 degree 2 poles (-59.469298, 88.188016) (-59.423338, 88.903316) (-60.270311, 89.829546) (-61.094139, 89.882478) knots 0 0 0 1 2 2 2
  spline S110 degree 2 poles (-61.094139, 89.882478) (-61.898235, 89.934143) (-62.854876, 89.153519) (-62.902737, 88.408621) knots 0 0 0 1 2 2 2
  spline S111 degree 2 poles (-62.902737, 88.408621) (-62.93158, 87.959708) (-62.673093, 87.125778) (-62.451656, 86.794528) knots 0 0 0 1 2 2 2
  line L135 (-62.451656, 86.794528) -> (-62.455143, 86.740264)
  line L136 (-62.455143, 86.740264) -> (-63.318436, 86.795732)
  spline S112 degree 2 poles (-63.318436, 86.795732) (-63.363825, 86.937346) (-63.490444, 87.356619) (-63.514199, 87.526563) knots 0 0 0 1 2 2 2
  spline S113 degree 2 poles (-63.514199, 87.526563) (-63.558182, 87.767156) (-63.593607, 88.140942) (-63.574589, 88.436928) knots 0 0 0 1 2 2 2
  spline S114 degree 2 poles (-63.505632, 84.487847) (-63.552344, 85.034558) (-63.387296, 86.006188) (-63.276319, 86.333192) knots 0 0 0 1 2 2 2
  line L137 (-63.276319, 86.333192) -> (-62.414387, 86.406836)
  line L138 (-62.414387, 86.406836) -> (-62.410179, 86.357583)
  spline S115 degree 2 poles (-62.410179, 86.357583) (-62.478884, 86.232642) (-62.639114, 85.901429) (-62.719821, 85.626624) knots 0 0 0 1 2 2 2
  spline S116 degree 2 poles (-62.719821, 85.626624) (-62.793624, 85.387138) (-62.883559, 84.813868) (-62.857468, 84.508497) knots 0 0 0 1 2 2 2
  spline S117 degree 2 poles (-62.857468, 84.508497) (-62.838531, 84.286857) (-62.707372, 83.796974) (-62.632822, 83.679312) knots 0 0 0 1 2 2 2
  spline S118 degree 2 poles (-62.632822, 83.679312) (-62.524933, 83.519846) (-62.300098, 83.385256) (-62.083384, 83.403772) knots 0 0 0 1 2 2 2
  spline S119 degree 2 poles (-62.083384, 83.403772) (-61.807566, 83.427339) (-61.562046, 83.805528) (-61.507181, 84.266654) knots 0 0 0 1 2 2 2
  spline S120 degree 2 poles (-61.507181, 84.266654) (-61.482928, 84.447333) (-61.437741, 85.021741) (-61.404183, 85.267711) knots 0 0 0 1 2 2 2
  spline S121 degree 2 poles (-61.404183, 85.267711) (-61.304942, 85.906274) (-60.722895, 86.526552) (-60.269765, 86.565268) knots 0 0 0 1 2 2 2
  spline S122 degree 2 poles (-60.269765, 86.565268) (-59.654099, 86.61787) (-58.785716, 85.570815) (-58.706601, 84.644853) knots 0 0 0 1 2 2 2
  spline S123 degree 2 poles (-58.706601, 84.644853) (-58.667885, 84.191723) (-58.776354, 83.254695) (-58.892677, 82.932196) knots 0 0 0 1 2 2 2
  line L139 (-58.892677, 82.932196) -> (-59.715207, 82.861918)
  line L140 (-59.715207, 82.861918) -> (-59.719415, 82.911172)
  spline S124 degree 2 poles (-59.719415, 82.911172) (-59.512877, 83.281069) (-59.316049, 84.171073) (-59.353502, 84.609427) knots 0 0 0 1 2 2 2
  spline S125 degree 2 poles (-59.353502, 84.609427) (-59.392218, 85.062557) (-59.765809, 85.66072) (-60.085956, 85.633367) knots 0 0 0 1 2 2 2
  spline S126 degree 2 poles (-60.085956, 85.633367) (-60.37655, 85.608538) (-60.625732, 85.215152) (-60.67946, 84.798775) knots 0 0 0 1 2 2 2
  spline S127 degree 2 poles (-60.67946, 84.798775) (-60.706113, 84.588123) (-60.751845, 84.078165) (-60.782037, 83.792792) knots 0 0 0 1 2 2 2
  spline S128 degree 2 poles (-60.782037, 83.792792) (-60.858334, 83.176035) (-61.392266, 82.515217) (-61.899575, 82.471872) knots 0 0 0 1 2 2 2
  spline S129 degree 2 poles (-61.899575, 82.471872) (-62.195095, 82.446622) (-62.741166, 82.682759) (-62.955979, 82.932315) knots 0 0 0 1 2 2 2
  spline S130 degree 2 poles (-62.955979, 82.932315) (-63.183167, 83.210581) (-63.458079, 83.931285) (-63.505632, 84.487847) knots 0 0 0 1 2 2 2
  point P0 (7, 0.000002)
  constraints: 1 coincident, 1 horizontal alignment, 3 other
extrude "Extrusion7" cut sketch "Sketch18" against normal blind 1 contours L0 L1 L2 L3 L4 L5 L6 L7 L8 L9 L10 L11 L12 | S0 S1 S2 S3 | L13 L14 S8 S9 S10 L15 L16 L17 S11 S12 S13 L18 L19 L20 | L21 L22 S14 S15 S16 L23 L24 L25 L26 L27 S17 S18 L28 | S19 L29 L30 L31 L32 L33 L34 L35 L36 L37 L38 L39 S20 S21 S22 L40 L41 S23 | L42 L43 L44 L45 L46 L47 L48 S24 S25 S26 L49 | S31 S32 S33 S34 | L53 L54 L55 L56 L57 L58 L59 L60 | S39 S40 S41 S42 S43 S44 L61 S45 S46 S47 L62 L63 S48 S49 S50 L64 L65 L66 | L68 L69 L70 L71 | L72 L73 L74 L75 L76 L77 L78 L79 L80 L81 L82 L83 | L84 L85 L86 L87 | S55 S56 S57 S58 L88 L89 S59 S60 S61 L90 L91 S62 S63 | S68 S69 S70 S71 S72 L99 L98 L93 L94 S73 S74 S75 S76 S77 L95 L96 S78 S79 | L99 L100 L101 L102 L103 L104 L105 L106 L107 S81 S82 S83 L108 L109 S84 S80 L97 L98 L93 S72 | S72 L93 L98 L99 | L110 S85 S86 L111 L112 L113 L114 L115 S87 S88 L116 | S89 S90 S91 S92 | L117 L118 S97 S98 S99 L119 L120 L121 L122 L123 S100 S101 L124 | L125 L126 L127 L128 | L129 L130 L131 L132 | S102 S103 S104 S105 S106 L133 L134 S107 S108 S109 S110 S111 L135 L136 S112 S113 | S114 L137 L138 S115 S116 S117 S118 S119 S120 S121 S122 S123 L139 L140 S124 S125 S126 S127 S128 S129 S130
body "Solid1"
